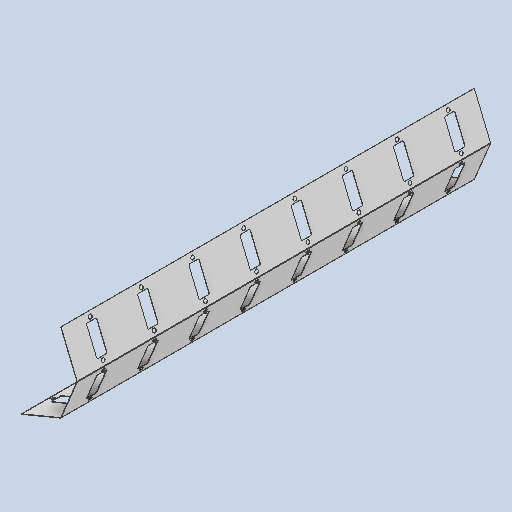
# Autodesk Inventor part: ДМФ 01 14 Барабан Лист прав брт
Saved by Autodesk Inventor 2024.2 (Build 282272000, 272)
## iProperties
Created: 2024-04-28
Part Number: ДМФ 01 14 Барабан Лист прав брт
Material: Generic
Document SubType Name: Sheet Metal
Designer: pokla
Density: 1 g/cm^3
Appearance: Default
Sheet Metal Rule: Default
Flat Pattern Width: 62.4873 cm
Flat Pattern Length: 202 cm
Flat Pattern Area: 12622.4 cm^2
Sheet Metal Width: 624,873 mm
Sheet Metal Length: 2020,000 mm
Sheet Metal Area: 1262242,781 mm^2
Author: pokla
Autodesk Inventor part; units mm, degrees
ref_plane "YZ Plane" through (0, 0, 0) normal (1, 0, 0) x (0, 1, 0)
ref_plane "XZ Plane" through (0, 0, 0) normal (0, 1, 0) x (-1, 0, 0)
ref_plane "XY Plane" through (0, 0, 0) normal (0, 0, 1) x (1, 0, 0)
sketch "Sketch2" plane through (0, 0, 0) normal (0, 0, 1) x (1, 0, 0)
  line L0 (0, 273.845227) -> (193.637817, 193.637817) construction
  line L1 (193.637817, 193.637817) -> (273.845227, 0) construction
  line L2 (273.845227, 0) -> (193.637817, -193.637817) construction
  line L3 (193.637817, -193.637817) -> (0, -273.845227) construction
  line L4 (0, -273.845227) -> (-193.637817, -193.637817) construction
  line L5 (-193.637817, -193.637817) -> (-273.845227, 0) construction
  line L6 (-273.845227, 0) -> (-193.637817, 193.637817) construction
  line L7 (-193.637817, 193.637817) -> (0, 273.845227) construction
  line L8 (193.982232, 192.806325) -> (273.211176, 1.530734)
  line L9 (273.211176, -1.530734) -> (194.271867, -192.107083)
  arc A0 (273.211176, -1.530734) -> (273.211176, 1.530734) centre (269.515658, 0) ccw
  line L10 (192.107083, -194.271867) -> (0.831492, -273.500812)
  arc A1 (192.107083, -194.271867) -> (194.271867, -192.107083) centre (190.576349, -190.576349) ccw
  point P0 (0, 0)
  point P1 (0, 0)
  dimension "d56" = 506
  dimension "d58" = 4
  dimension "d69" = 0.9
  dimension "d70" = 4
  dimension "d71" = 0.9
  measures "d56" distance between parallel lines of L6 L2
  measures "d58" radius of A0
  measures "d69" distance of L3.end L10.end
  measures "d70" radius of A1
  measures "d71" distance of L0.end L8.start
contour flange "Contour Flange2" sketch "Sketch2" thickness 2 bend radius 2 width 2020 along (0, 0, -1) mid plane no both sides no wall seen from (233.596704, 97.168529, 0) lies toward (-0.9238795, -0.3826834, 0) curves L8 A0 L9 A1 L10
bend "Bend2"
corner "Corner2"
sketch "Sketch10" plane through (194.271867, -192.107083, 0) normal (0.9238795, -0.3826834, 0) x (0, 0, -1)
  line L0 (1110, 170.639177) -> (1160, 170.639177)
  line L1 (1160, 170.639177) -> (1160, 35.639177)
  line L2 (1160, 35.639177) -> (1110, 35.639177)
  line L3 (1110, 35.639177) -> (1110, 170.639177)
  line L4 (1110, 103.139177) -> (1160, 103.139177) construction
  line L5 (2020, 206.278354) -> (2020, 0) construction
  line L6 (2020, 206.278354) -> (0, 206.278354) construction
  line L7 (1135, 185.639177) -> (1135, 20.639177) construction
  line L8 (1130.381198, 177.639177) -> (1125.762396, 185.639177)
  line L9 (1125.762396, 185.639177) -> (1130.381198, 193.639177)
  line L10 (1130.381198, 193.639177) -> (1139.618802, 193.639177)
  line L11 (1139.618802, 193.639177) -> (1144.237604, 185.639177)
  line L12 (1144.237604, 185.639177) -> (1139.618802, 177.639177)
  line L13 (1139.618802, 177.639177) -> (1130.381198, 177.639177)
  line L14 (1139.618802, 28.639177) -> (1144.237604, 20.639177)
  line L15 (1144.237604, 20.639177) -> (1139.618802, 12.639177)
  line L16 (1139.618802, 12.639177) -> (1130.381198, 12.639177)
  line L17 (1130.381198, 12.639177) -> (1125.762396, 20.639177)
  line L18 (1125.762396, 20.639177) -> (1130.381198, 28.639177)
  line L19 (1130.381198, 28.639177) -> (1139.618802, 28.639177)
  point P0 (0, 103.139177)
  point P1 (1135, 170.639177)
  point P2 (2020, 103.139177)
  point P3 (1010, 206.278354)
  point P4 (1010, 206.278354)
  point P5 (1135, 103.139177)
  point P6 (1135, 177.639177)
  point P7 (1135, 28.639177)
  dimension "d107" = 135
  dimension "d108" = 50
  dimension "d118" = 125
  dimension "d125" = 165
  dimension "d126" = 16
  dimension "d127" = 16
  constraints: 36 end point, 10 midpoint, 2 coincident, 2 parallel, 2 point on line, 1 horizontal, 1 horizontal alignment, 1 perpendicular, 1 vertical, 26 other
  measures "d107" distance of L0.end L1.end
  measures "d108" distance of L0.start L0.end
  measures "d118" horizontal distance of point (1010, 206.278) point (1135, 170.639)
  measures "d125" distance of L7.start L7.end
  measures "d126" distance between parallel lines of L13 L10
  measures "d127" distance between parallel lines of L16 L19
extrude "Extrusion4" cut sketch "Sketch10" against normal up to surface (2 mm away)
fillet "Fillet1" radius 5 4 edges at (258.6488, -34.0744, -1160) (258.6488, -34.0744, -1110) (206.9865, -158.7981, -1110) (206.9865, -158.7981, -1160)
pattern_circular "Circular Pattern1" count 3 over 90 about axis through (0, 0, -10) along (0, 0, 1) of "Extrusion4", "Fillet1" both ways yes
pattern_linear "Rectangular Pattern2" count 8 spacing 250 along (0, 0, 1) of "Extrusion4", "Fillet1", "Circular Pattern1" first direction both ways yes
chamfer "Corner Chamfer1" distance 2 angle 45 1 edges at (193.0584, 192.4236, -2020)
equation "\"d118\" = Барабан_Отступ_окна_от_середины"
equation "\"d56\" = Барабан_габарит_по_кассетам"
equation "\"d58\" = BendRadius + Thickness"
equation "\"d69\" = Барабан_отступ_развертки"
equation "\"d70\" = BendRadius + Thickness"
equation "\"d71\" = Барабан_отступ_развертки"
equation "\"d107\" = Барабан_Длина_окна"
equation "\"d108\" = Барабан_Ширина_окна"
equation "\"d25\" = Thickness"
equation "\"d26\" = BendReliefWidth"
equation "\"d27\" = BendReliefDepth"
equation "\"d28\" = MinimumRemnant"
equation "\"d29\" = TransitionRadius"
equation "\"d30\" = Барабан_длина_листа"
equation "\"d31\" = BendRadius"
equation "\"d33\" = CornerReliefSize"
equation "\"d34\" = GapSize"
equation "\"d35\" = JacobiRadiusSize"
equation "\"BendRadius\" = Thickness"
equation "\"BendReliefWidth\" = Thickness"
equation "\"BendReliefDepth\" = 0.5 * Thickness"
equation "\"CornerReliefSize\" = 4 * Thickness"
equation "\"MinimumRemnant\" = 2 * Thickness"
equation "\"TransitionRadius\" = BendRadius"
equation "\"JacobiRadiusSize\" = BendRadius"
equation "\"GapSize\" = Thickness"
equation "\"Барабан_габарит_по_кассетам\" = 506"
equation "\"Thickness\" = 2"
equation "\"Барабан_отступ_развертки\" = 0.9"
equation "\"Барабан_Длина_окна\" = 135"
equation "\"Барабан_Ширина_окна\" = 50"
equation "\"Барабан_длина_листа\" = 2020"
equation "\"Барабан_Отступ_окна_от_середины\" = 125"
body "Solid2"
